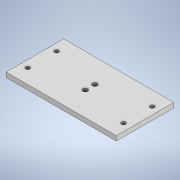
# Autodesk Inventor part: AjusteBalancin
Saved by Autodesk Inventor 2022 (Build 260153000, 153)
## iProperties
Created: 2022-02-28
Part Number: AjusteBalancin
Material: Generic
Document SubType Name: Modeling
Designer: hurta
Density: 1 g/cm^3
Appearance: Default
Author: hurta
Autodesk Inventor part; units mm, degrees
ref_plane "YZ Plane" through (0, 0, 0) normal (1, 0, 0) x (0, 1, 0)
ref_plane "XZ Plane" through (0, 0, 0) normal (0, 1, 0) x (-1, 0, 0)
ref_plane "XY Plane" through (0, 0, 0) normal (0, 0, 1) x (1, 0, 0)
sketch "Sketch1" plane through (0, 0, 0) normal (0, 1, 0) x (-1, 0, 0)
  line L0 (57.5, -30) -> (-57.5, -30)
  line L1 (-57.5, -30) -> (-57.5, 30)
  line L2 (-57.5, 30) -> (57.5, 30)
  line L3 (57.5, 30) -> (57.5, -30)
  line L4 (57.5, -30) -> (-57.5, 30) construction
  line L5 (-57.5, -30) -> (57.5, 30) construction
  point P0 (0, 0)
  dimension "d0" = 115
  dimension "d1" = 60
  constraints: 12 end point, 2 midpoint, 2 parallel, 1 horizontal, 1 perpendicular
  measures "d0" distance of L1.end L2.end
  measures "d1" distance of L0.end L1.end
extrude "Extrusion1" add sketch "Sketch1" along normal blind 5
sketch "Sketch2" plane through (0, 5, 0) normal (0, 1, 0) x (1, 0, 0)
  line L0 (57.5, 30) -> (-57.5, 30) projected
  line L1 (-57.5, 30) -> (-57.5, -30) projected
  line L2 (-57.5, -30) -> (57.5, -30) projected
  line L3 (57.5, -30) -> (57.5, 30) projected
  point P0 (0, 0)
  point P1 (-50, -15)
  point P2 (-50, 15)
  point P3 (50, -15)
  point P4 (50, 15)
  dimension "d4" = 15
  dimension "d5" = 7.5
  dimension "d6" = 15
  dimension "d7" = 7.5
  constraints: 2 horizontal alignment, 2 vertical alignment
  measures "d4" distance from line of point (-50, 15) L0
  measures "d5" distance from line of L1 point (-50, 15)
  measures "d6" distance from line of point (-50, -15) L2
  measures "d7" distance from line of L3 point (50, -15)
hole "Hole1" at (-50, 5, 15) at (-50, 5, -15) at (50, 5, 15) at (50, 5, -15) direction (0, -1, 0) diameter 4.5 end through all
sketch "Sketch3" plane through (0, 5, 0) normal (0, 1, 0) x (1, 0, 0)
  point P0 (0, 0)
  point P1 (0, -5)
  point P2 (0, 5)
  dimension "d15" = 5
  dimension "d16" = 5
  constraints: 2 vertical alignment
  measures "d15" distance of point (0, 5) point (0, 0)
  measures "d16" distance of point (0, 0) point (0, -5)
hole "Hole2" at (0, 5, 5) at (0, 5, -5) direction (0, -1, 0) diameter 5.2 end through all clearance for "Hex Head Bolt" size "M5" standard "Ansi Metric M Profile"
equation "\"d6\" = d4"
equation "\"d7\" = d5"
body "Solid1"
